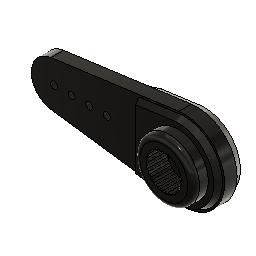
Servo Horn (Autodesk Fusion 360 design; units mm, degrees)
Autodesk Fusion 360 part; units mm, degrees
sketch "Sketch1" plane through (0, 0, 0) normal (0, 0, 1) x (1, 0, 0)
  circle A0 centre (0, 0) radius 3
  circle A1 centre (0, 0) radius 6.875
  circle A2 centre (-13.25, 0) radius 0.6
  circle A3 centre (-16.25, 0) radius 0.6
  circle A4 centre (-19.25, 0) radius 0.6
  circle A5 centre (-22.25, 0) radius 0.6
  circle A6 centre (-22.25, 0) radius 3.875
  line L0 (0, 0) -> (-22.25, 0) construction
  line L1 (-22.25, 0) -> (-26.125, 0) construction
  line L2 (0, 0) -> (6.875, 0) construction
  line L3 (-0.927, 6.8122) -> (-22.7725, 3.8396)
  line L4 (-22.7725, -3.8396) -> (-0.927, -6.8122)
  circle A7 centre (0, 0) radius 1.275
  line L5 (-8.125, 5.8328) -> (-8.125, -5.8328)
  dimension "d1" = 1.2
  dimension "d2" = 3
  dimension "d3" = 3
  dimension "d4" = 3
  dimension "d5" = 33
  dimension "d6" = 13.75
  dimension "d7" = 6
  dimension "d8" = 7.75
  dimension "d11" = 2.55
  dimension "d13" = 15
  measures "d1" diameter of A2
  measures "d4" distance of A0.centre
  measures "d5" distance of A0.centre
  measures "d6" diameter of A1
  measures "d7" diameter of A0
  measures "d8" diameter of A6
  measures "d11" diameter of A7
  measures "d13" distance of L5
extrude "Extrude1" add sketch "Sketch1" along normal blind 2.15 contours A0 | A1 | A1 L3 L4 L5 | A6 L3 L4 L5 | A6
ref_plane "WorkPlane1" through (-8.9829, 0, -1.3) normal (0, 0, -1) x (-1, 0, 0)
sketch "Sketch2" plane through (-8.9829, 0, -1.3) normal (0, 0, -1) x (1, 0, 0)
  line L0 (0.8579, -5.8328) -> (0.8579, 5.8328)
  line L1 (-13.7895, 3.8396) -> (8.056, 6.8122)
  line L2 (8.056, -6.8122) -> (-13.7895, -3.8396)
  circle A0 centre (8.9829, 0) radius 6.875
  circle A1 centre (8.9829, 0) radius 3
  line L3 (0.8579, -5.8328) -> (8.056, -6.8122)
  line L4 (0.8579, 5.8328) -> (8.056, 6.8122)
  circle A2 centre (8.9829, 0) radius 4.5
  arc A3 (8.056, -6.8122) -> (8.056, 6.8122) centre (8.9829, 0) ccw
  line L5 (1.6079, 5.1779) -> (8.1571, 6.0691)
  arc A4 (8.1571, -6.0691) -> (8.1571, 6.0691) centre (8.9829, 0) ccw
  line L6 (1.6079, -5.1779) -> (8.1571, -6.0691)
  line L7 (1.6079, -5.1779) -> (1.6079, 5.1779)
  dimension "d14" = 9
  dimension "d15" = 0.75
  measures "d14" diameter of A2
  measures "d15" distance of L4
loft "Loft1" add profiles "Sketch1", "Sketch2" section 1 contours A1 | A1 L3 L4 L5 section 2 contours A0 L5 L6 L7 | A0 L5 A4 L6
sketch "Sketch3" plane through (0, 0, 2.15) normal (0, 0, 1) x (1, 0, 0)
  circle A0 centre (-16.25, 0) radius 0.6
  circle A1 centre (-22.25, 0) radius 0.6
  circle A2 centre (-19.25, 0) radius 0.6
  circle A3 centre (-13.25, 0) radius 0.6
  circle A4 centre (0, 0) radius 1.275
  line L0 (-22.7725, -3.8396) -> (-0.927, -6.8122)
  arc A5 (-0.927, -6.8122) -> (-0.927, 6.8122) centre (0, 0) ccw
  line L1 (-0.927, 6.8122) -> (-22.7725, 3.8396)
  arc A6 (-22.7725, 3.8396) -> (-22.7725, -3.8396) centre (-22.25, 0) ccw
  line L2 (-8.125, 5.8328) -> (-8.125, -5.8328)
  line L3 (-8.125, -5.8328) -> (-0.927, -6.8122)
  arc A7 (-0.927, -6.8122) -> (-0.927, 6.8122) centre (0, 0) ccw
  line L4 (-0.927, 6.8122) -> (-8.125, 5.8328)
  arc A8 (-0.8798, -6.4654) -> (-0.8798, 6.4654) centre (0, 0) ccw
  line L5 (-0.8798, 6.4654) -> (-7.775, 5.5272)
  line L6 (-7.775, 5.5272) -> (-7.775, -5.5272)
  line L7 (-7.775, -5.5272) -> (-0.8798, -6.4654)
  circle A9 centre (0, 0) radius 1.275
  dimension "d16" = 0.35
ref_plane "WorkPlane2" through (-0.0156, 0, 3.15) normal (0, 0, 1) x (1, 0, 0)
sketch "Sketch4" plane through (-0.0156, 0, 3.15) normal (0, 0, 1) x (1, 0, 0)
  arc A0 (-0.8642, -6.4654) -> (-0.8642, 6.4654) centre (0.0156, 0) ccw
  line L0 (-0.8642, 6.4654) -> (-7.7594, 5.5272)
  line L1 (-7.7594, 5.5272) -> (-7.7594, -5.5272)
  line L2 (-7.7594, -5.5272) -> (-0.8642, -6.4654)
  arc A1 (-0.7967, -5.97) -> (-0.7967, 5.97) centre (0.0156, 0) ccw
  line L3 (-0.7967, 5.97) -> (-7.2594, 5.0906)
  line L4 (-7.2594, 5.0906) -> (-7.2594, -5.0906)
  line L5 (-7.2594, -5.0906) -> (-0.7967, -5.97)
  circle A2 centre (0.0156, 0) radius 1.275
  dimension "d18" = 0.5
loft "Loft3" add profiles "Sketch3", "Sketch4" section 1 contours A8 L5 L6 L7 section 2 contours A1 L3 L4 L5
sketch "Sketch5" plane through (0, 0, 3.15) normal (0, 0, 1) x (1, 0, 0)
  spline S0 degree 3 poles (-7.275, -5.0906) (-5.1404, -5.381) (-3.0059, -5.6715) (-0.8713, -5.962) (-0.8517, -5.9646) (-0.832, -5.9673) (-0.8124, -5.97) (0.0679, -6.0898) (0.9745, -6.0117) (1.8213, -5.7431) (3.2775, -5.2813) (4.5422, -4.243) (5.2787, -2.9045) (5.8265, -1.9089) (6.0845, -0.7559) (6.0131, 0.3782) (5.9601, 1.2219) (5.7269, 2.0537) (5.3338, 2.8021) (4.756, 3.9019) (3.8289, 4.815) (2.7203, 5.3759) (1.6385, 5.9233) (0.389, 6.1335) (-0.8124, 5.97) (-0.832, 5.9673) (-0.8517, 5.9646) (-0.8713, 5.962) (-3.0059, 5.6715) (-5.1404, 5.381) (-7.275, 5.0906) knots 0 0 0 0 0.19233 0.19233 0.19233 0.1941 0.1941 0.1941 0.273412 0.273412 0.273412 0.409806 0.409806 0.409806 0.511263 0.511263 0.511263 0.586733 0.586733 0.586733 0.697655 0.697655 0.697655 0.8059 0.8059 0.8059 0.80767 0.80767 0.80767 1 1 1 1
  line L0 (-7.275, 5.0906) -> (-7.275, -5.0906)
  circle A0 centre (0, 0) radius 5.1
  spline S1 degree 3 poles (-2.0506, 2.0802) (-2.0155, 2.0662) (-1.9764, 2.0587) (-1.9089, 2.0601) (-1.8773, 2.065) (-1.815, 2.0871) (-1.7844, 2.1044) (-1.7328, 2.1471) (-1.7101, 2.174) (-1.6767, 2.231) (-1.6659, 2.2611) (-1.6518, 2.3272) (-1.6519, 2.367) (-1.6592, 2.404) knots -0.084316 -0.084316 -0.084316 -0.084316 -0.069983 -0.069983 -0.059928 -0.059928 -0.049872 -0.049872 -0.039817 -0.039817 -0.029761 -0.029761 -0.015429 -0.015429 -0.015429 -0.015429
  arc A1 (2.8817, -0.4777) -> (2.9099, -0.254) centre (0, 0) ccw
  arc A2 (2.2951, -1.8068) -> (2.4276, -1.6245) centre (0, 0) ccw
  arc A3 (-1.4688, 2.5248) -> (-1.6592, 2.404) centre (0, 0) ccw
  spline S2 degree 3 poles (2.8817, -0.4777) (2.845, -0.4869) (2.809, -0.5038) (2.7552, -0.5446) (2.7325, -0.5672) (2.6952, -0.6217) (2.6806, -0.6536) (2.6639, -0.7186) (2.6613, -0.7536) (2.6678, -0.8193) (2.6768, -0.8501) (2.7043, -0.9118) (2.7277, -0.9439) (2.7553, -0.9697) knots -0.084316 -0.084316 -0.084316 -0.084316 -0.069983 -0.069983 -0.059928 -0.059928 -0.049872 -0.049872 -0.039817 -0.039817 -0.029761 -0.029761 -0.015429 -0.015429 -0.015429 -0.015429
  arc A4 (2.6724, -1.1793) -> (2.7553, -0.9697) centre (0, 0) ccw
  arc A5 (-0.7948, 2.8108) -> (-1.0092, 2.7411) centre (0, 0) ccw
  spline S3 degree 3 poles (2.6724, -1.1793) (2.6346, -1.1791) (2.5955, -1.1865) (2.5332, -1.2127) (2.5056, -1.229) (2.4559, -1.2724) (2.4338, -1.2997) (2.4015, -1.3585) (2.3903, -1.3918) (2.3802, -1.4571) (2.3813, -1.4891) (2.3925, -1.5557) (2.4072, -1.5926) (2.4276, -1.6245) knots -0.084316 -0.084316 -0.084316 -0.084316 -0.069983 -0.069983 -0.059928 -0.059928 -0.049872 -0.049872 -0.039817 -0.039817 -0.029761 -0.029761 -0.015429 -0.015429 -0.015429 -0.015429
  spline S4 degree 3 poles (-1.4688, 2.5248) (-1.4383, 2.5025) (-1.4024, 2.4855) (-1.3366, 2.4701) (-1.3047, 2.467) (-1.2389, 2.4729) (-1.205, 2.4821) (-1.1444, 2.5106) (-1.1157, 2.5309) (-1.0692, 2.5778) (-1.0512, 2.6044) (-1.0212, 2.6649) (-1.0114, 2.7034) (-1.0092, 2.7411) knots -0.084316 -0.084316 -0.084316 -0.084316 -0.069983 -0.069983 -0.059928 -0.059928 -0.049872 -0.049872 -0.039817 -0.039817 -0.029761 -0.029761 -0.015429 -0.015429 -0.015429 -0.015429
  circle A6 centre (0, 0) radius 2.7305
  circle A7 centre (0, 0) radius 1.778
  arc A8 (1.3448, 2.593) -> (1.1408, 2.689) centre (0, 0) ccw
  circle A9 centre (0, 0) radius 2.7305
  arc A10 (1.7737, -2.3208) -> (1.9474, -2.1771) centre (0, 0) ccw
  spline S5 degree 3 poles (0.6577, 2.846) (0.6646, 2.8088) (0.6791, 2.7718) (0.7165, 2.7156) (0.7377, 2.6915) (0.7897, 2.6508) (0.8207, 2.6342) (0.8844, 2.6135) (0.9192, 2.6087) (0.9852, 2.6111) (1.0165, 2.6181) (1.0798, 2.6417) (1.1133, 2.663) (1.1408, 2.689) knots -0.084316 -0.084316 -0.084316 -0.084316 -0.069983 -0.069983 -0.059928 -0.059928 -0.049872 -0.049872 -0.039817 -0.039817 -0.029761 -0.029761 -0.015429 -0.015429 -0.015429 -0.015429
  spline S6 degree 3 poles (1.7737, -2.3208) (1.7406, -2.3025) (1.7028, -2.2901) (1.6357, -2.2831) (1.6036, -2.284) (1.5391, -2.2982) (1.5066, -2.3115) (1.45, -2.3474) (1.4241, -2.3711) (1.3839, -2.4235) (1.3694, -2.4521) (1.3471, -2.5159) (1.3422, -2.5553) (1.3448, -2.593) knots -0.084316 -0.084316 -0.084316 -0.084316 -0.069983 -0.069983 -0.059928 -0.059928 -0.049872 -0.049872 -0.039817 -0.039817 -0.029761 -0.029761 -0.015429 -0.015429 -0.015429 -0.015429
  spline S7 degree 3 poles (2.4276, 1.6245) (2.4072, 1.5926) (2.3925, 1.5557) (2.3813, 1.4891) (2.3802, 1.4571) (2.3903, 1.3918) (2.4015, 1.3585) (2.4338, 1.2997) (2.4559, 1.2724) (2.5056, 1.229) (2.5332, 1.2127) (2.5955, 1.1865) (2.6346, 1.1791) (2.6724, 1.1793) knots -0.084316 -0.084316 -0.084316 -0.084316 -0.069983 -0.069983 -0.059928 -0.059928 -0.049872 -0.049872 -0.039817 -0.039817 -0.029761 -0.029761 -0.015429 -0.015429 -0.015429 -0.015429
  spline S8 degree 3 poles (2.2951, -1.8068) (2.2586, -1.7973) (2.2189, -1.7947) (2.1521, -1.8046) (2.1213, -1.8135) (2.0623, -1.8432) (2.0341, -1.8642) (1.9882, -1.913) (1.9691, -1.9425) (1.9431, -2.0032) (1.9362, -2.0345) (1.9305, -2.1018) (1.9355, -2.1412) (1.9474, -2.1771) knots -0.084316 -0.084316 -0.084316 -0.084316 -0.069983 -0.069983 -0.059928 -0.059928 -0.049872 -0.049872 -0.039817 -0.039817 -0.029761 -0.029761 -0.015429 -0.015429 -0.015429 -0.015429
  spline S9 degree 3 poles (-1.6592, -2.404) (-1.6519, -2.367) (-1.6518, -2.3272) (-1.6659, -2.2611) (-1.6767, -2.231) (-1.7101, -2.174) (-1.7328, -2.1471) (-1.7844, -2.1044) (-1.815, -2.0871) (-1.8773, -2.065) (-1.9089, -2.0601) (-1.9764, -2.0587) (-2.0155, -2.0662) (-2.0506, -2.0802) knots -0.084316 -0.084316 -0.084316 -0.084316 -0.069983 -0.069983 -0.059928 -0.059928 -0.049872 -0.049872 -0.039817 -0.039817 -0.029761 -0.029761 -0.015429 -0.015429 -0.015429 -0.015429
  arc A11 (-2.5035, 1.5049) -> (-2.6121, 1.3074) centre (0, 0) ccw
  arc A12 (1.1408, -2.689) -> (1.3448, -2.593) centre (0, 0) ccw
  arc A13 (-1.0092, -2.7411) -> (-0.7948, -2.8108) centre (0, 0) ccw
  spline S10 degree 3 poles (-1.0092, -2.7411) (-1.0114, -2.7034) (-1.0212, -2.6649) (-1.0512, -2.6044) (-1.0692, -2.5778) (-1.1157, -2.5309) (-1.1444, -2.5106) (-1.205, -2.4821) (-1.2389, -2.4729) (-1.3047, -2.467) (-1.3366, -2.4701) (-1.4024, -2.4855) (-1.4383, -2.5025) (-1.4688, -2.5248) knots -0.084316 -0.084316 -0.084316 -0.084316 -0.069983 -0.069983 -0.059928 -0.059928 -0.049872 -0.049872 -0.039817 -0.039817 -0.029761 -0.029761 -0.015429 -0.015429 -0.015429 -0.015429
  spline S11 degree 3 poles (2.7553, 0.9697) (2.7277, 0.9439) (2.7043, 0.9118) (2.6768, 0.8501) (2.6678, 0.8193) (2.6613, 0.7536) (2.6639, 0.7186) (2.6806, 0.6536) (2.6952, 0.6217) (2.7325, 0.5672) (2.7552, 0.5446) (2.809, 0.5038) (2.845, 0.4869) (2.8817, 0.4777) knots -0.084316 -0.084316 -0.084316 -0.084316 -0.069983 -0.069983 -0.059928 -0.059928 -0.049872 -0.049872 -0.039817 -0.039817 -0.029761 -0.029761 -0.015429 -0.015429 -0.015429 -0.015429
  spline S12 degree 3 poles (1.1408, -2.689) (1.1133, -2.663) (1.0798, -2.6417) (1.0165, -2.6181) (0.9852, -2.6111) (0.9192, -2.6087) (0.8844, -2.6135) (0.8207, -2.6342) (0.7897, -2.6508) (0.7377, -2.6915) (0.7165, -2.7156) (0.6791, -2.7718) (0.6646, -2.8088) (0.6577, -2.846) knots -0.084316 -0.084316 -0.084316 -0.084316 -0.069983 -0.069983 -0.059928 -0.059928 -0.049872 -0.049872 -0.039817 -0.039817 -0.029761 -0.029761 -0.015429 -0.015429 -0.015429 -0.015429
  spline S13 degree 3 poles (1.3448, 2.593) (1.3422, 2.5553) (1.3471, 2.5159) (1.3694, 2.4521) (1.3839, 2.4235) (1.4241, 2.3711) (1.45, 2.3474) (1.5066, 2.3115) (1.5391, 2.2982) (1.6036, 2.284) (1.6357, 2.2831) (1.7028, 2.2901) (1.7406, 2.3025) (1.7737, 2.3208) knots -0.084316 -0.084316 -0.084316 -0.084316 -0.069983 -0.069983 -0.059928 -0.059928 -0.049872 -0.049872 -0.039817 -0.039817 -0.029761 -0.029761 -0.015429 -0.015429 -0.015429 -0.015429
  arc A14 (-1.6592, -2.404) -> (-1.4688, -2.5248) centre (0, 0) ccw
  arc A15 (2.7553, 0.9697) -> (2.6724, 1.1793) centre (0, 0) ccw
  arc A16 (-0.0708, 2.9201) -> (-0.2958, 2.906) centre (0, 0) ccw
  spline S14 degree 3 poles (-0.7948, 2.8108) (-0.7708, 2.7816) (-0.7402, 2.7562) (-0.6803, 2.7249) (-0.6502, 2.714) (-0.585, 2.7034) (-0.5499, 2.7038) (-0.484, 2.7163) (-0.4512, 2.7289) (-0.3945, 2.7628) (-0.3705, 2.784) (-0.3264, 2.8351) (-0.3073, 2.87) (-0.2958, 2.906) knots -0.084316 -0.084316 -0.084316 -0.084316 -0.069983 -0.069983 -0.059928 -0.059928 -0.049872 -0.049872 -0.039817 -0.039817 -0.029761 -0.029761 -0.015429 -0.015429 -0.015429 -0.015429
  spline S15 degree 3 poles (-0.0708, 2.9201) (-0.0548, 2.8859) (-0.0315, 2.8537) (0.0187, 2.8085) (0.0452, 2.7904) (0.1057, 2.7639) (0.1398, 2.7556) (0.2067, 2.7514) (0.2416, 2.7554) (0.3049, 2.7741) (0.3335, 2.7887) (0.3889, 2.8272) (0.4161, 2.8562) (0.4362, 2.8882) knots -0.084316 -0.084316 -0.084316 -0.084316 -0.069983 -0.069983 -0.059928 -0.059928 -0.049872 -0.049872 -0.039817 -0.039817 -0.029761 -0.029761 -0.015429 -0.015429 -0.015429 -0.015429
  arc A17 (-0.2958, -2.906) -> (-0.0708, -2.9201) centre (0, 0) ccw
  arc A18 (-2.2049, -1.9159) -> (-2.0506, -2.0802) centre (0, 0) ccw
  spline S16 degree 3 poles (-2.2049, -1.9159) (-2.1887, -1.8818) (-2.1787, -1.8433) (-2.1759, -1.7758) (-2.1788, -1.7439) (-2.197, -1.6804) (-2.2123, -1.6488) (-2.2517, -1.5945) (-2.277, -1.5702) (-2.3318, -1.5333) (-2.3613, -1.5206) (-2.4263, -1.5025) (-2.466, -1.5) (-2.5035, -1.5049) knots -0.084316 -0.084316 -0.084316 -0.084316 -0.069983 -0.069983 -0.059928 -0.059928 -0.049872 -0.049872 -0.039817 -0.039817 -0.029761 -0.029761 -0.015429 -0.015429 -0.015429 -0.015429
  arc A19 (2.9099, 0.254) -> (2.8817, 0.4777) centre (0, 0) ccw
  spline S17 degree 3 poles (-0.2958, -2.906) (-0.3073, -2.87) (-0.3264, -2.8351) (-0.3705, -2.784) (-0.3945, -2.7628) (-0.4512, -2.7289) (-0.484, -2.7163) (-0.5499, -2.7038) (-0.585, -2.7034) (-0.6502, -2.714) (-0.6803, -2.7249) (-0.7402, -2.7562) (-0.7708, -2.7816) (-0.7948, -2.8108) knots -0.084316 -0.084316 -0.084316 -0.084316 -0.069983 -0.069983 -0.059928 -0.059928 -0.049872 -0.049872 -0.039817 -0.039817 -0.029761 -0.029761 -0.015429 -0.015429 -0.015429 -0.015429
  spline S18 degree 3 poles (2.9099, 0.254) (2.8767, 0.2359) (2.8461, 0.2106) (2.8041, 0.1577) (2.7878, 0.1301) (2.7651, 0.0681) (2.7589, 0.0335) (2.7589, -0.0335) (2.7651, -0.0681) (2.7878, -0.1301) (2.8041, -0.1577) (2.8461, -0.2106) (2.8767, -0.2359) (2.9099, -0.254) knots -0.084316 -0.084316 -0.084316 -0.084316 -0.069983 -0.069983 -0.059928 -0.059928 -0.049872 -0.049872 -0.039817 -0.039817 -0.029761 -0.029761 -0.015429 -0.015429 -0.015429 -0.015429
  arc A20 (0.4362, -2.8882) -> (0.6577, -2.846) centre (0, 0) ccw
  arc A21 (-2.0506, 2.0802) -> (-2.2049, 1.9159) centre (0, 0) ccw
  arc A22 (1.9474, 2.1771) -> (1.7737, 2.3208) centre (0, 0) ccw
  spline S19 degree 3 poles (1.9474, 2.1771) (1.9355, 2.1412) (1.9305, 2.1018) (1.9362, 2.0345) (1.9431, 2.0032) (1.9691, 1.9425) (1.9882, 1.913) (2.0341, 1.8642) (2.0623, 1.8432) (2.1213, 1.8135) (2.1521, 1.8046) (2.2189, 1.7947) (2.2586, 1.7973) (2.2951, 1.8068) knots -0.084316 -0.084316 -0.084316 -0.084316 -0.069983 -0.069983 -0.059928 -0.059928 -0.049872 -0.049872 -0.039817 -0.039817 -0.029761 -0.029761 -0.015429 -0.015429 -0.015429 -0.015429
  arc A23 (2.4276, 1.6245) -> (2.2951, 1.8068) centre (0, 0) ccw
  arc A24 (-2.6121, -1.3074) -> (-2.5035, -1.5049) centre (0, 0) ccw
  spline S20 degree 3 poles (0.4362, -2.8882) (0.4161, -2.8562) (0.3889, -2.8272) (0.3335, -2.7887) (0.3049, -2.7741) (0.2416, -2.7554) (0.2067, -2.7514) (0.1398, -2.7556) (0.1057, -2.7639) (0.0452, -2.7904) (0.0187, -2.8085) (-0.0315, -2.8537) (-0.0548, -2.8859) (-0.0708, -2.9201) knots -0.084316 -0.084316 -0.084316 -0.084316 -0.069983 -0.069983 -0.059928 -0.059928 -0.049872 -0.049872 -0.039817 -0.039817 -0.029761 -0.029761 -0.015429 -0.015429 -0.015429 -0.015429
  arc A25 (-2.8552, -0.6167) -> (-2.7991, -0.8351) centre (0, 0) ccw
  spline S21 degree 3 poles (-2.7991, 0.8351) (-2.7616, 0.8396) (-2.7237, 0.8519) (-2.6652, 0.8856) (-2.6399, 0.9052) (-2.596, 0.9546) (-2.5775, 0.9845) (-2.5528, 1.0468) (-2.5459, 1.0812) (-2.5441, 1.1472) (-2.5491, 1.1789) (-2.5686, 1.2436) (-2.5879, 1.2784) (-2.6121, 1.3074) knots -0.084316 -0.084316 -0.084316 -0.084316 -0.069983 -0.069983 -0.059928 -0.059928 -0.049872 -0.049872 -0.039817 -0.039817 -0.029761 -0.029761 -0.015429 -0.015429 -0.015429 -0.015429
  spline S22 degree 3 poles (-2.5035, 1.5049) (-2.466, 1.5) (-2.4263, 1.5025) (-2.3613, 1.5206) (-2.3318, 1.5333) (-2.277, 1.5702) (-2.2517, 1.5945) (-2.2123, 1.6488) (-2.197, 1.6804) (-2.1788, 1.7439) (-2.1759, 1.7758) (-2.1787, 1.8433) (-2.1887, 1.8818) (-2.2049, 1.9159) knots -0.084316 -0.084316 -0.084316 -0.084316 -0.069983 -0.069983 -0.059928 -0.059928 -0.049872 -0.049872 -0.039817 -0.039817 -0.029761 -0.029761 -0.015429 -0.015429 -0.015429 -0.015429
  spline S23 degree 3 poles (-2.8552, -0.6167) (-2.8245, -0.5946) (-2.7972, -0.5657) (-2.7622, -0.5079) (-2.7495, -0.4785) (-2.7348, -0.4141) (-2.7329, -0.379) (-2.7413, -0.3125) (-2.7518, -0.279) (-2.7821, -0.2203) (-2.8018, -0.195) (-2.85, -0.1477) (-2.8836, -0.1265) (-2.9188, -0.1127) knots -0.084316 -0.084316 -0.084316 -0.084316 -0.069983 -0.069983 -0.059928 -0.059928 -0.049872 -0.049872 -0.039817 -0.039817 -0.029761 -0.029761 -0.015429 -0.015429 -0.015429 -0.015429
  spline S24 degree 3 poles (-2.6121, -1.3074) (-2.5879, -1.2784) (-2.5686, -1.2436) (-2.5491, -1.1789) (-2.5441, -1.1472) (-2.5459, -1.0812) (-2.5528, -1.0468) (-2.5775, -0.9845) (-2.596, -0.9546) (-2.6399, -0.9052) (-2.6652, -0.8856) (-2.7237, -0.8519) (-2.7616, -0.8396) (-2.7991, -0.8351) knots -0.084316 -0.084316 -0.084316 -0.084316 -0.069983 -0.069983 -0.059928 -0.059928 -0.049872 -0.049872 -0.039817 -0.039817 -0.029761 -0.029761 -0.015429 -0.015429 -0.015429 -0.015429
  arc A26 (-2.7991, 0.8351) -> (-2.8552, 0.6167) centre (0, 0) ccw
  arc A27 (0.6577, 2.846) -> (0.4362, 2.8882) centre (0, 0) ccw
  spline S25 degree 3 poles (-2.9188, 0.1127) (-2.8836, 0.1265) (-2.85, 0.1477) (-2.8018, 0.195) (-2.7821, 0.2203) (-2.7518, 0.279) (-2.7413, 0.3125) (-2.7329, 0.379) (-2.7348, 0.4141) (-2.7495, 0.4785) (-2.7622, 0.5079) (-2.7972, 0.5657) (-2.8245, 0.5946) (-2.8552, 0.6167) knots -0.084316 -0.084316 -0.084316 -0.084316 -0.069983 -0.069983 -0.059928 -0.059928 -0.049872 -0.049872 -0.039817 -0.039817 -0.029761 -0.029761 -0.015429 -0.015429 -0.015429 -0.015429
  arc A28 (-2.9188, 0.1127) -> (-2.9188, -0.1127) centre (0, 0) ccw
  spline S26 degree 3 poles (-0.0074, 3.021) (0.0017, 3.0014) (0.0108, 2.9819) (0.0199, 2.9623) (0.0302, 2.9401) (0.0458, 2.9186) (0.0649, 2.9014) (0.078, 2.8897) (0.0962, 2.8772) (0.1155, 2.8688) (0.1346, 2.8604) (0.1584, 2.8546) (0.1795, 2.8533) (0.2007, 2.8519) (0.225, 2.8547) (0.2449, 2.8606) (0.2652, 2.8666) (0.2848, 2.8767) (0.2993, 2.8867) (0.3204, 2.9013) (0.3385, 2.9207) (0.3516, 2.9415) (0.363, 2.9597) (0.3745, 2.978) (0.386, 2.9962) knots -0.092492 -0.092492 -0.092492 -0.092492 -0.084316 -0.084316 -0.084316 -0.069983 -0.069983 -0.069983 -0.059928 -0.059928 -0.059928 -0.049872 -0.049872 -0.049872 -0.039817 -0.039817 -0.039817 -0.029761 -0.029761 -0.029761 -0.015429 -0.015429 -0.015429 -0.007252 -0.007252 -0.007252 -0.007252
  arc A29 (0.7441, 2.9279) -> (0.386, 2.9962) centre (0, 0) ccw
  spline S27 degree 3 poles (0.7441, 2.9279) (0.7481, 2.9067) (0.752, 2.8855) (0.756, 2.8643) (0.7604, 2.8402) (0.7702, 2.8155) (0.7844, 2.7941) (0.7941, 2.7795) (0.8087, 2.7629) (0.8253, 2.7499) (0.8417, 2.7371) (0.8633, 2.7255) (0.8834, 2.719) (0.9036, 2.7124) (0.9278, 2.7091) (0.9487, 2.7098) (0.9697, 2.7106) (0.9913, 2.7154) (1.0078, 2.7216) (1.0318, 2.7305) (1.0542, 2.7448) (1.072, 2.7616) (1.0877, 2.7765) (1.1033, 2.7913) (1.119, 2.8061) knots -0.092492 -0.092492 -0.092492 -0.092492 -0.084316 -0.084316 -0.084316 -0.069983 -0.069983 -0.069983 -0.059928 -0.059928 -0.059928 -0.049872 -0.049872 -0.049872 -0.039817 -0.039817 -0.039817 -0.029761 -0.029761 -0.029761 -0.015429 -0.015429 -0.015429 -0.007252 -0.007252 -0.007252 -0.007252
  arc A30 (1.4489, 2.6509) -> (1.119, 2.8061) centre (0, 0) ccw
  spline S28 degree 3 poles (1.4489, 2.6509) (1.4474, 2.6294) (1.446, 2.6079) (1.4445, 2.5863) (1.4429, 2.5619) (1.4462, 2.5355) (1.4546, 2.5113) (1.4604, 2.4947) (1.4704, 2.475) (1.4833, 2.4583) (1.496, 2.4417) (1.514, 2.4252) (1.5319, 2.4139) (1.5498, 2.4025) (1.5724, 2.3932) (1.5928, 2.3888) (1.6134, 2.3843) (1.6354, 2.3836) (1.6529, 2.3854) (1.6785, 2.3881) (1.7037, 2.3964) (1.7251, 2.4083) (1.744, 2.4187) (1.7628, 2.4292) (1.7817, 2.4397) knots -0.092492 -0.092492 -0.092492 -0.092492 -0.084316 -0.084316 -0.084316 -0.069983 -0.069983 -0.069983 -0.059928 -0.059928 -0.059928 -0.049872 -0.049872 -0.049872 -0.039817 -0.039817 -0.039817 -0.029761 -0.029761 -0.029761 -0.015429 -0.015429 -0.015429 -0.007252 -0.007252 -0.007252 -0.007252
  arc A31 (2.0626, 2.2073) -> (1.7817, 2.4397) centre (0, 0) ccw
  spline S29 degree 3 poles (2.0626, 2.2073) (2.0558, 2.1868) (2.0491, 2.1663) (2.0424, 2.1459) (2.0347, 2.1226) (2.0313, 2.0962) (2.0335, 2.0706) (2.0349, 2.0531) (2.0397, 2.0316) (2.048, 2.0122) (2.0562, 1.993) (2.0696, 1.9725) (2.084, 1.9571) (2.0985, 1.9416) (2.1182, 1.927) (2.1368, 1.9176) (2.1556, 1.9081) (2.1768, 1.902) (2.1942, 1.8994) (2.2196, 1.8957) (2.2461, 1.8974) (2.2699, 1.9036) (2.2907, 1.909) (2.3116, 1.9145) (2.3324, 1.9199) knots -0.092492 -0.092492 -0.092492 -0.092492 -0.084316 -0.084316 -0.084316 -0.069983 -0.069983 -0.069983 -0.059928 -0.059928 -0.059928 -0.049872 -0.049872 -0.049872 -0.039817 -0.039817 -0.039817 -0.029761 -0.029761 -0.029761 -0.015429 -0.015429 -0.015429 -0.007252 -0.007252 -0.007252 -0.007252
  arc A32 (2.5467, 1.625) -> (2.3324, 1.9199) centre (0, 0) ccw
  spline S30 degree 3 poles (2.5467, 1.625) (2.5351, 1.6068) (2.5235, 1.5887) (2.5118, 1.5705) (2.4986, 1.5499) (2.4888, 1.5252) (2.4845, 1.4999) (2.4816, 1.4825) (2.4809, 1.4605) (2.4841, 1.4396) (2.4873, 1.419) (2.4951, 1.3958) (2.5053, 1.3773) (2.5155, 1.3587) (2.5309, 1.3397) (2.5466, 1.326) (2.5624, 1.3121) (2.5815, 1.3009) (2.5977, 1.2941) (2.6213, 1.2841) (2.6474, 1.2792) (2.6719, 1.2793) (2.6935, 1.2794) (2.7151, 1.2795) (2.7366, 1.2796) knots -0.092492 -0.092492 -0.092492 -0.092492 -0.084316 -0.084316 -0.084316 -0.069983 -0.069983 -0.069983 -0.059928 -0.059928 -0.059928 -0.049872 -0.049872 -0.049872 -0.039817 -0.039817 -0.039817 -0.029761 -0.029761 -0.029761 -0.015429 -0.015429 -0.015429 -0.007252 -0.007252 -0.007252 -0.007252
  arc A33 (2.8708, 0.9406) -> (2.7366, 1.2796) centre (0, 0) ccw
  spline S31 degree 3 poles (2.8708, 0.9406) (2.8551, 0.9259) (2.8393, 0.9112) (2.8235, 0.8965) (2.8056, 0.8798) (2.7899, 0.8583) (2.7795, 0.8349) (2.7723, 0.8188) (2.7661, 0.7976) (2.7641, 0.7766) (2.762, 0.7559) (2.7638, 0.7315) (2.7691, 0.711) (2.7744, 0.6905) (2.7845, 0.6682) (2.7963, 0.651) (2.8082, 0.6336) (2.8239, 0.618) (2.8379, 0.6074) (2.8583, 0.5919) (2.8824, 0.5806) (2.9061, 0.5746) (2.9271, 0.5693) (2.948, 0.5641) (2.9689, 0.5588) knots -0.092492 -0.092492 -0.092492 -0.092492 -0.084316 -0.084316 -0.084316 -0.069983 -0.069983 -0.069983 -0.059928 -0.059928 -0.059928 -0.049872 -0.049872 -0.049872 -0.039817 -0.039817 -0.039817 -0.029761 -0.029761 -0.029761 -0.015429 -0.015429 -0.015429 -0.007252 -0.007252 -0.007252 -0.007252
  arc A34 (3.0146, 0.1971) -> (2.9689, 0.5588) centre (0, 0) ccw
  spline S32 degree 3 poles (3.0146, 0.1971) (2.9956, 0.1868) (2.9767, 0.1765) (2.9577, 0.1662) (2.9362, 0.1545) (2.9157, 0.1376) (2.8998, 0.1174) (2.8889, 0.1036) (2.8776, 0.0846) (2.8704, 0.0648) (2.8632, 0.0453) (2.8589, 0.0212) (2.8589, 0) (2.8589, -0.0212) (2.8632, -0.0453) (2.8704, -0.0648) (2.8776, -0.0846) (2.8889, -0.1036) (2.8998, -0.1174) (2.9157, -0.1376) (2.9362, -0.1545) (2.9577, -0.1662) (2.9767, -0.1765) (2.9956, -0.1868) (3.0146, -0.1971) knots -0.092492 -0.092492 -0.092492 -0.092492 -0.084316 -0.084316 -0.084316 -0.069983 -0.069983 -0.069983 -0.059928 -0.059928 -0.059928 -0.049872 -0.049872 -0.049872 -0.039817 -0.039817 -0.039817 -0.029761 -0.029761 -0.029761 -0.015429 -0.015429 -0.015429 -0.007252 -0.007252 -0.007252 -0.007252
  arc A35 (2.9689, -0.5588) -> (3.0146, -0.1971) centre (0, 0) ccw
  spline S33 degree 3 poles (2.9689, -0.5588) (2.948, -0.5641) (2.9271, -0.5693) (2.9061, -0.5746) (2.8824, -0.5806) (2.8583, -0.5919) (2.8379, -0.6074) (2.8239, -0.618) (2.8082, -0.6336) (2.7963, -0.651) (2.7845, -0.6682) (2.7744, -0.6905) (2.7691, -0.711) (2.7638, -0.7315) (2.762, -0.7559) (2.7641, -0.7766) (2.7661, -0.7976) (2.7723, -0.8188) (2.7795, -0.8349) (2.7899, -0.8583) (2.8056, -0.8798) (2.8235, -0.8965) (2.8393, -0.9112) (2.8551, -0.9259) (2.8708, -0.9406) knots -0.092492 -0.092492 -0.092492 -0.092492 -0.084316 -0.084316 -0.084316 -0.069983 -0.069983 -0.069983 -0.059928 -0.059928 -0.059928 -0.049872 -0.049872 -0.049872 -0.039817 -0.039817 -0.039817 -0.029761 -0.029761 -0.029761 -0.015429 -0.015429 -0.015429 -0.007252 -0.007252 -0.007252 -0.007252
  arc A36 (2.7366, -1.2796) -> (2.8708, -0.9406) centre (0, 0) ccw
  spline S34 degree 3 poles (2.7366, -1.2796) (2.7151, -1.2795) (2.6935, -1.2794) (2.6719, -1.2793) (2.6474, -1.2792) (2.6213, -1.2841) (2.5977, -1.2941) (2.5815, -1.3009) (2.5624, -1.3121) (2.5466, -1.326) (2.5309, -1.3397) (2.5155, -1.3587) (2.5053, -1.3773) (2.4951, -1.3958) (2.4873, -1.419) (2.4841, -1.4396) (2.4809, -1.4605) (2.4816, -1.4825) (2.4845, -1.4999) (2.4888, -1.5252) (2.4986, -1.5499) (2.5118, -1.5705) (2.5235, -1.5887) (2.5351, -1.6068) (2.5467, -1.625) knots -0.092492 -0.092492 -0.092492 -0.092492 -0.084316 -0.084316 -0.084316 -0.069983 -0.069983 -0.069983 -0.059928 -0.059928 -0.059928 -0.049872 -0.049872 -0.049872 -0.039817 -0.039817 -0.039817 -0.029761 -0.029761 -0.029761 -0.015429 -0.015429 -0.015429 -0.007252 -0.007252 -0.007252 -0.007252
  arc A37 (2.3324, -1.9199) -> (2.5467, -1.625) centre (0, 0) ccw
  spline S35 degree 3 poles (2.3324, -1.9199) (2.3116, -1.9145) (2.2907, -1.909) (2.2699, -1.9036) (2.2461, -1.8974) (2.2196, -1.8957) (2.1942, -1.8994) (2.1768, -1.902) (2.1556, -1.9081) (2.1368, -1.9176) (2.1182, -1.927) (2.0985, -1.9416) (2.084, -1.9571) (2.0696, -1.9725) (2.0562, -1.993) (2.048, -2.0122) (2.0397, -2.0316) (2.0349, -2.0531) (2.0335, -2.0706) (2.0313, -2.0962) (2.0347, -2.1226) (2.0424, -2.1459) (2.0491, -2.1663) (2.0558, -2.1868) (2.0626, -2.2073) knots -0.092492 -0.092492 -0.092492 -0.092492 -0.084316 -0.084316 -0.084316 -0.069983 -0.069983 -0.069983 -0.059928 -0.059928 -0.059928 -0.049872 -0.049872 -0.049872 -0.039817 -0.039817 -0.039817 -0.029761 -0.029761 -0.029761 -0.015429 -0.015429 -0.015429 -0.007252 -0.007252 -0.007252 -0.007252
  arc A38 (1.7817, -2.4397) -> (2.0626, -2.2073) centre (0, 0) ccw
  spline S36 degree 3 poles (1.7817, -2.4397) (1.7628, -2.4292) (1.744, -2.4187) (1.7251, -2.4083) (1.7037, -2.3964) (1.6785, -2.3881) (1.6529, -2.3854) (1.6354, -2.3836) (1.6134, -2.3843) (1.5928, -2.3888) (1.5724, -2.3932) (1.5498, -2.4025) (1.5319, -2.4139) (1.514, -2.4252) (1.496, -2.4417) (1.4833, -2.4583) (1.4704, -2.475) (1.4604, -2.4947) (1.4546, -2.5113) (1.4462, -2.5355) (1.4429, -2.5619) (1.4445, -2.5863) (1.446, -2.6079) (1.4474, -2.6294) (1.4489, -2.6509) knots -0.092492 -0.092492 -0.092492 -0.092492 -0.084316 -0.084316 -0.084316 -0.069983 -0.069983 -0.069983 -0.059928 -0.059928 -0.059928 -0.049872 -0.049872 -0.049872 -0.039817 -0.039817 -0.039817 -0.029761 -0.029761 -0.029761 -0.015429 -0.015429 -0.015429 -0.007252 -0.007252 -0.007252 -0.007252
  arc A39 (1.119, -2.8061) -> (1.4489, -2.6509) centre (0, 0) ccw
  spline S37 degree 3 poles (1.119, -2.8061) (1.1033, -2.7913) (1.0877, -2.7765) (1.072, -2.7616) (1.0542, -2.7448) (1.0318, -2.7305) (1.0078, -2.7216) (0.9913, -2.7154) (0.9697, -2.7106) (0.9487, -2.7098) (0.9278, -2.7091) (0.9036, -2.7124) (0.8834, -2.719) (0.8633, -2.7255) (0.8417, -2.7371) (0.8253, -2.7499) (0.8087, -2.7629) (0.7941, -2.7795) (0.7844, -2.7941) (0.7702, -2.8155) (0.7604, -2.8402) (0.756, -2.8643) (0.752, -2.8855) (0.7481, -2.9067) (0.7441, -2.9279) knots -0.092492 -0.092492 -0.092492 -0.092492 -0.084316 -0.084316 -0.084316 -0.069983 -0.069983 -0.069983 -0.059928 -0.059928 -0.059928 -0.049872 -0.049872 -0.049872 -0.039817 -0.039817 -0.039817 -0.029761 -0.029761 -0.029761 -0.015429 -0.015429 -0.015429 -0.007252 -0.007252 -0.007252 -0.007252
  arc A40 (0.386, -2.9962) -> (0.7441, -2.9279) centre (0, 0) ccw
  spline S38 degree 3 poles (0.386, -2.9962) (0.3745, -2.978) (0.363, -2.9597) (0.3516, -2.9415) (0.3385, -2.9207) (0.3204, -2.9013) (0.2993, -2.8867) (0.2848, -2.8767) (0.2652, -2.8666) (0.2449, -2.8606) (0.225, -2.8547) (0.2007, -2.8519) (0.1795, -2.8533) (0.1584, -2.8546) (0.1346, -2.8604) (0.1155, -2.8688) (0.0962, -2.8772) (0.078, -2.8897) (0.0649, -2.9014) (0.0458, -2.9186) (0.0302, -2.9401) (0.0199, -2.9623) (0.0108, -2.9819) (0.0017, -3.0014) (-0.0074, -3.021) knots -0.092492 -0.092492 -0.092492 -0.092492 -0.084316 -0.084316 -0.084316 -0.069983 -0.069983 -0.069983 -0.059928 -0.059928 -0.059928 -0.049872 -0.049872 -0.049872 -0.039817 -0.039817 -0.039817 -0.029761 -0.029761 -0.029761 -0.015429 -0.015429 -0.015429 -0.007252 -0.007252 -0.007252 -0.007252
  arc A41 (-0.3713, -2.9981) -> (-0.0074, -3.021) centre (0, 0) ccw
  spline S39 degree 3 poles (-0.3713, -2.9981) (-0.3778, -2.9776) (-0.3844, -2.957) (-0.391, -2.9365) (-0.3985, -2.9132) (-0.4112, -2.8899) (-0.428, -2.8704) (-0.4395, -2.8571) (-0.4561, -2.8425) (-0.4742, -2.8317) (-0.4921, -2.821) (-0.5149, -2.8122) (-0.5357, -2.8083) (-0.5565, -2.8043) (-0.581, -2.804) (-0.6015, -2.8074) (-0.6224, -2.8108) (-0.6431, -2.8183) (-0.6587, -2.8264) (-0.6815, -2.8383) (-0.7019, -2.8553) (-0.7175, -2.8742) (-0.7311, -2.8909) (-0.7448, -2.9076) (-0.7585, -2.9242) knots -0.092492 -0.092492 -0.092492 -0.092492 -0.084316 -0.084316 -0.084316 -0.069983 -0.069983 -0.069983 -0.059928 -0.059928 -0.059928 -0.049872 -0.049872 -0.049872 -0.039817 -0.039817 -0.039817 -0.029761 -0.029761 -0.029761 -0.015429 -0.015429 -0.015429 -0.007252 -0.007252 -0.007252 -0.007252
  arc A42 (-1.1052, -2.8116) -> (-0.7585, -2.9242) centre (0, 0) ccw
  spline S40 degree 3 poles (-1.1052, -2.8116) (-1.1065, -2.7901) (-1.1077, -2.7685) (-1.109, -2.747) (-1.1104, -2.7225) (-1.117, -2.6968) (-1.1284, -2.6738) (-1.1362, -2.658) (-1.1486, -2.6398) (-1.1635, -2.6248) (-1.1781, -2.61) (-1.1981, -2.5958) (-1.2173, -2.5868) (-1.2364, -2.5778) (-1.2601, -2.5714) (-1.2808, -2.5696) (-1.3018, -2.5677) (-1.3238, -2.5698) (-1.3409, -2.5738) (-1.3659, -2.5797) (-1.3899, -2.591) (-1.4097, -2.6055) (-1.4271, -2.6182) (-1.4445, -2.631) (-1.4619, -2.6437) knots -0.092492 -0.092492 -0.092492 -0.092492 -0.084316 -0.084316 -0.084316 -0.069983 -0.069983 -0.069983 -0.059928 -0.059928 -0.059928 -0.049872 -0.049872 -0.049872 -0.039817 -0.039817 -0.039817 -0.029761 -0.029761 -0.029761 -0.015429 -0.015429 -0.015429 -0.007252 -0.007252 -0.007252 -0.007252
  arc A43 (-1.7697, -2.4484) -> (-1.4619, -2.6437) centre (0, 0) ccw
  spline S41 degree 3 poles (-1.7697, -2.4484) (-1.7656, -2.4272) (-1.7614, -2.4061) (-1.7573, -2.3849) (-1.7526, -2.3609) (-1.7526, -2.3343) (-1.7579, -2.3092) (-1.7616, -2.292) (-1.769, -2.2712) (-1.7797, -2.253) (-1.7902, -2.235) (-1.806, -2.2163) (-1.8223, -2.2028) (-1.8387, -2.1893) (-1.86, -2.1773) (-1.8796, -2.1703) (-1.8995, -2.1633) (-1.9213, -2.1598) (-1.9389, -2.1595) (-1.9645, -2.1589) (-1.9906, -2.1639) (-2.0134, -2.1731) (-2.0334, -2.1811) (-2.0534, -2.1891) (-2.0734, -2.1971) knots -0.092492 -0.092492 -0.092492 -0.092492 -0.084316 -0.084316 -0.084316 -0.069983 -0.069983 -0.069983 -0.059928 -0.059928 -0.059928 -0.049872 -0.049872 -0.049872 -0.039817 -0.039817 -0.039817 -0.029761 -0.029761 -0.029761 -0.015429 -0.015429 -0.015429 -0.007252 -0.007252 -0.007252 -0.007252
  arc A44 (-2.323, -1.9314) -> (-2.0734, -2.1971) centre (0, 0) ccw
  spline S42 degree 3 poles (-2.323, -1.9314) (-2.3137, -1.9119) (-2.3045, -1.8924) (-2.2952, -1.873) (-2.2847, -1.8508) (-2.278, -1.8251) (-2.2769, -1.7994) (-2.2762, -1.7819) (-2.2783, -1.7599) (-2.2841, -1.7396) (-2.2898, -1.7196) (-2.3005, -1.6976) (-2.3129, -1.6804) (-2.3253, -1.6633) (-2.343, -1.6463) (-2.3603, -1.6347) (-2.3778, -1.6229) (-2.3981, -1.6142) (-2.415, -1.6094) (-2.4397, -1.6025) (-2.4662, -1.6009) (-2.4905, -1.6041) (-2.5119, -1.6069) (-2.5333, -1.6097) (-2.5547, -1.6125) knots -0.092492 -0.092492 -0.092492 -0.092492 -0.084316 -0.084316 -0.084316 -0.069983 -0.069983 -0.069983 -0.059928 -0.059928 -0.059928 -0.049872 -0.049872 -0.049872 -0.039817 -0.039817 -0.039817 -0.029761 -0.029761 -0.029761 -0.015429 -0.015429 -0.015429 -0.007252 -0.007252 -0.007252 -0.007252
  arc A45 (-2.7303, -1.293) -> (-2.5547, -1.6125) centre (0, 0) ccw
  spline S43 degree 3 poles (-2.7303, -1.293) (-2.7165, -1.2764) (-2.7027, -1.2599) (-2.6889, -1.2433) (-2.6732, -1.2245) (-2.6603, -1.2012) (-2.6529, -1.1767) (-2.6478, -1.1598) (-2.6444, -1.138) (-2.6449, -1.1169) (-2.6455, -1.0961) (-2.6503, -1.0721) (-2.6581, -1.0524) (-2.6659, -1.0327) (-2.6788, -1.0119) (-2.6927, -0.9964) (-2.7067, -0.9806) (-2.7241, -0.9671) (-2.7394, -0.9583) (-2.7616, -0.9455) (-2.7869, -0.9373) (-2.8112, -0.9343) (-2.8326, -0.9317) (-2.854, -0.9291) (-2.8754, -0.9265) knots -0.092492 -0.092492 -0.092492 -0.092492 -0.084316 -0.084316 -0.084316 -0.069983 -0.069983 -0.069983 -0.059928 -0.059928 -0.059928 -0.049872 -0.049872 -0.049872 -0.039817 -0.039817 -0.039817 -0.029761 -0.029761 -0.029761 -0.015429 -0.015429 -0.015429 -0.007252 -0.007252 -0.007252 -0.007252
  arc A46 (-2.9661, -0.5734) -> (-2.8754, -0.9265) centre (0, 0) ccw
  spline S44 degree 3 poles (-2.9661, -0.5734) (-2.9486, -0.5608) (-2.9311, -0.5482) (-2.9136, -0.5356) (-2.8937, -0.5212) (-2.8755, -0.5019) (-2.8622, -0.4799) (-2.8531, -0.4649) (-2.8443, -0.4446) (-2.8396, -0.4241) (-2.835, -0.4038) (-2.8337, -0.3793) (-2.8364, -0.3583) (-2.839, -0.3373) (-2.8463, -0.314) (-2.8559, -0.2954) (-2.8655, -0.2767) (-2.8791, -0.2592) (-2.8916, -0.2469) (-2.91, -0.229) (-2.9324, -0.2148) (-2.9553, -0.2058) (-2.9753, -0.198) (-2.9954, -0.1901) (-3.0155, -0.1823) knots -0.092492 -0.092492 -0.092492 -0.092492 -0.084316 -0.084316 -0.084316 -0.069983 -0.069983 -0.069983 -0.059928 -0.059928 -0.059928 -0.049872 -0.049872 -0.049872 -0.039817 -0.039817 -0.039817 -0.029761 -0.029761 -0.029761 -0.015429 -0.015429 -0.015429 -0.007252 -0.007252 -0.007252 -0.007252
  arc A47 (-3.0155, 0.1823) -> (-3.0155, -0.1823) centre (0, 0) ccw
  spline S45 degree 3 poles (-3.0155, 0.1823) (-2.9954, 0.1901) (-2.9753, 0.198) (-2.9553, 0.2058) (-2.9324, 0.2148) (-2.91, 0.229) (-2.8916, 0.2469) (-2.8791, 0.2592) (-2.8655, 0.2767) (-2.8559, 0.2954) (-2.8463, 0.314) (-2.839, 0.3373) (-2.8364, 0.3583) (-2.8337, 0.3793) (-2.835, 0.4038) (-2.8396, 0.4241) (-2.8443, 0.4446) (-2.8531, 0.4649) (-2.8622, 0.4799) (-2.8755, 0.5019) (-2.8937, 0.5212) (-2.9136, 0.5356) (-2.9311, 0.5482) (-2.9486, 0.5608) (-2.9661, 0.5734) knots -0.092492 -0.092492 -0.092492 -0.092492 -0.084316 -0.084316 -0.084316 -0.069983 -0.069983 -0.069983 -0.059928 -0.059928 -0.059928 -0.049872 -0.049872 -0.049872 -0.039817 -0.039817 -0.039817 -0.029761 -0.029761 -0.029761 -0.015429 -0.015429 -0.015429 -0.007252 -0.007252 -0.007252 -0.007252
  arc A48 (-2.8754, 0.9265) -> (-2.9661, 0.5734) centre (0, 0) ccw
  spline S46 degree 3 poles (-2.8754, 0.9265) (-2.854, 0.9291) (-2.8326, 0.9317) (-2.8112, 0.9343) (-2.7869, 0.9373) (-2.7616, 0.9455) (-2.7394, 0.9583) (-2.7241, 0.9671) (-2.7067, 0.9806) (-2.6927, 0.9964) (-2.6788, 1.0119) (-2.6659, 1.0327) (-2.6581, 1.0524) (-2.6503, 1.0721) (-2.6455, 1.0961) (-2.6449, 1.1169) (-2.6444, 1.138) (-2.6478, 1.1598) (-2.6529, 1.1767) (-2.6603, 1.2012) (-2.6732, 1.2245) (-2.6889, 1.2433) (-2.7027, 1.2599) (-2.7165, 1.2764) (-2.7303, 1.293) knots -0.092492 -0.092492 -0.092492 -0.092492 -0.084316 -0.084316 -0.084316 -0.069983 -0.069983 -0.069983 -0.059928 -0.059928 -0.059928 -0.049872 -0.049872 -0.049872 -0.039817 -0.039817 -0.039817 -0.029761 -0.029761 -0.029761 -0.015429 -0.015429 -0.015429 -0.007252 -0.007252 -0.007252 -0.007252
  arc A49 (-2.5547, 1.6125) -> (-2.7303, 1.293) centre (0, 0) ccw
  spline S47 degree 3 poles (-2.5547, 1.6125) (-2.5333, 1.6097) (-2.5119, 1.6069) (-2.4905, 1.6041) (-2.4662, 1.6009) (-2.4397, 1.6025) (-2.415, 1.6094) (-2.3981, 1.6142) (-2.3778, 1.6229) (-2.3603, 1.6347) (-2.343, 1.6463) (-2.3253, 1.6633) (-2.3129, 1.6804) (-2.3005, 1.6976) (-2.2898, 1.7196) (-2.2841, 1.7396) (-2.2783, 1.7599) (-2.2762, 1.7819) (-2.2769, 1.7994) (-2.278, 1.8251) (-2.2847, 1.8508) (-2.2952, 1.873) (-2.3045, 1.8924) (-2.3137, 1.9119) (-2.323, 1.9314) knots -0.092492 -0.092492 -0.092492 -0.092492 -0.084316 -0.084316 -0.084316 -0.069983 -0.069983 -0.069983 -0.059928 -0.059928 -0.059928 -0.049872 -0.049872 -0.049872 -0.039817 -0.039817 -0.039817 -0.029761 -0.029761 -0.029761 -0.015429 -0.015429 -0.015429 -0.007252 -0.007252 -0.007252 -0.007252
  arc A50 (-2.0734, 2.1971) -> (-2.323, 1.9314) centre (0, 0) ccw
  spline S48 degree 3 poles (-2.0734, 2.1971) (-2.0534, 2.1891) (-2.0334, 2.1811) (-2.0134, 2.1731) (-1.9906, 2.1639) (-1.9645, 2.1589) (-1.9389, 2.1595) (-1.9213, 2.1598) (-1.8995, 2.1633) (-1.8796, 2.1703) (-1.86, 2.1773) (-1.8387, 2.1893) (-1.8223, 2.2028) (-1.806, 2.2163) (-1.7902, 2.235) (-1.7797, 2.253) (-1.769, 2.2712) (-1.7616, 2.292) (-1.7579, 2.3092) (-1.7526, 2.3343) (-1.7526, 2.3609) (-1.7573, 2.3849) (-1.7614, 2.4061) (-1.7656, 2.4272) (-1.7697, 2.4484) knots -0.092492 -0.092492 -0.092492 -0.092492 -0.084316 -0.084316 -0.084316 -0.069983 -0.069983 -0.069983 -0.059928 -0.059928 -0.059928 -0.049872 -0.049872 -0.049872 -0.039817 -0.039817 -0.039817 -0.029761 -0.029761 -0.029761 -0.015429 -0.015429 -0.015429 -0.007252 -0.007252 -0.007252 -0.007252
  arc A51 (-1.4619, 2.6437) -> (-1.7697, 2.4484) centre (0, 0) ccw
  spline S49 degree 3 poles (-1.4619, 2.6437) (-1.4445, 2.631) (-1.4271, 2.6182) (-1.4097, 2.6055) (-1.3899, 2.591) (-1.3659, 2.5797) (-1.3409, 2.5738) (-1.3238, 2.5698) (-1.3018, 2.5677) (-1.2808, 2.5696) (-1.2601, 2.5714) (-1.2364, 2.5778) (-1.2173, 2.5868) (-1.1981, 2.5958) (-1.1781, 2.61) (-1.1635, 2.6248) (-1.1486, 2.6398) (-1.1362, 2.658) (-1.1284, 2.6738) (-1.117, 2.6968) (-1.1104, 2.7225) (-1.109, 2.747) (-1.1077, 2.7685) (-1.1065, 2.7901) (-1.1052, 2.8116) knots -0.092492 -0.092492 -0.092492 -0.092492 -0.084316 -0.084316 -0.084316 -0.069983 -0.069983 -0.069983 -0.059928 -0.059928 -0.059928 -0.049872 -0.049872 -0.049872 -0.039817 -0.039817 -0.039817 -0.029761 -0.029761 -0.029761 -0.015429 -0.015429 -0.015429 -0.007252 -0.007252 -0.007252 -0.007252
  arc A52 (-0.7585, 2.9242) -> (-1.1052, 2.8116) centre (0, 0) ccw
  spline S50 degree 3 poles (-0.7585, 2.9242) (-0.7448, 2.9076) (-0.7311, 2.8909) (-0.7175, 2.8742) (-0.7019, 2.8553) (-0.6815, 2.8383) (-0.6587, 2.8264) (-0.6431, 2.8183) (-0.6224, 2.8108) (-0.6015, 2.8074) (-0.581, 2.804) (-0.5565, 2.8043) (-0.5357, 2.8083) (-0.5149, 2.8122) (-0.4921, 2.821) (-0.4742, 2.8317) (-0.4561, 2.8425) (-0.4395, 2.8571) (-0.428, 2.8704) (-0.4112, 2.8899) (-0.3985, 2.9132) (-0.391, 2.9365) (-0.3844, 2.957) (-0.3778, 2.9776) (-0.3713, 2.9981) knots -0.092492 -0.092492 -0.092492 -0.092492 -0.084316 -0.084316 -0.084316 -0.069983 -0.069983 -0.069983 -0.059928 -0.059928 -0.059928 -0.049872 -0.049872 -0.049872 -0.039817 -0.039817 -0.039817 -0.029761 -0.029761 -0.029761 -0.015429 -0.015429 -0.015429 -0.007252 -0.007252 -0.007252 -0.007252
  arc A53 (-0.0074, 3.021) -> (-0.3713, 2.9981) centre (0, 0) ccw
  dimension "d19" = 10.2
  dimension "d20" = 0.1
  measures "d19" diameter of A0
  measures "d20" distance of S15
extrude "Extrude2" add sketch "Sketch5" along normal blind 2.5 contours A0
extrude "Extrude3" cut 1 faces at (0.714, -0.4483, 3.15) along direction (0, 0, -1) blind 1
ref_plane "WorkPlane3" through (-0.5948, 0.0222, 0.95) normal (0, 0, -1) x (-1, 0, 0)
sketch "Sketch6" plane through (-0.5948, 0.0222, 0.95) normal (0, 0, -1) x (1, 0, 0)
  circle A0 centre (0.5948, 0.0222) radius 3
  circle A1 centre (0.5948, 0.0222) radius 1.275
  dimension "d26" = 6
  measures "d26" diameter of A0
loft "Loft4" cut profiles "Sketch6", "Sketch2" section 1 contours A0 | A1 section 2 contours A2
fillet "Fillet1" radius 1 1 edges at (-4.7549, -1.8442, 5.65)
